Autodesk Fusion 360 part; units mm, degrees
(part 7 of 7)
  line L820 (63.0336, -72.9522) -> (63.1893, -72.6515)
  line L821 (63.1893, -72.6515) -> (63.3708, -72.7431)
  line L822 (63.3708, -72.7431) -> (63.5541, -72.8309)
  line L823 (63.5541, -72.8309) -> (63.7392, -72.9149)
  line L824 (63.7392, -72.9149) -> (63.9261, -72.995)
  line L825 (63.9261, -72.995) -> (63.7958, -73.3076)
  line L826 (63.7958, -73.3076) -> (63.771, -73.385)
  line L827 (63.771, -73.385) -> (63.7515, -73.4645)
  line L828 (63.7515, -73.4645) -> (63.7355, -73.5455)
  line L829 (63.7355, -73.5455) -> (63.7225, -73.6277)
  line L830 (63.7225, -73.6277) -> (63.7121, -73.7109)
  line L831 (63.7121, -73.7109) -> (63.704, -73.795)
  line L832 (63.704, -73.795) -> (63.6981, -73.8799)
  line L833 (63.6981, -73.8799) -> (63.6944, -73.9656)
  line L834 (63.6944, -73.9656) -> (63.6926, -74.0521)
  line L835 (63.6926, -74.0521) -> (63.6927, -74.1391)
  line L836 (63.6927, -74.1391) -> (63.6947, -74.2268)
  line L837 (63.6947, -74.2268) -> (63.6986, -74.3151)
  line L838 (63.6986, -74.3151) -> (63.8305, -74.365)
  line L839 (63.8305, -74.365) -> (63.9631, -74.4133)
  line L840 (63.9631, -74.4133) -> (64.0963, -74.4599)
  line L841 (64.0963, -74.4599) -> (64.156, -74.3947)
  line L842 (64.156, -74.3947) -> (64.2139, -74.3288)
  line L843 (64.2139, -74.3288) -> (64.2699, -74.2622)
  line L844 (64.2699, -74.2622) -> (64.3241, -74.1949)
  line L845 (64.3241, -74.1949) -> (64.3763, -74.1268)
  line L846 (64.3763, -74.1268) -> (64.4264, -74.058)
  line L847 (64.4264, -74.058) -> (64.4743, -73.9883)
  line L848 (64.4743, -73.9883) -> (64.5198, -73.9179)
  line L849 (64.5198, -73.9179) -> (64.5627, -73.8466)
  line L850 (64.5627, -73.8466) -> (64.6025, -73.7743)
  line L851 (64.6025, -73.7743) -> (64.6387, -73.7008)
  line L852 (64.6387, -73.7008) -> (64.6694, -73.6256)
  line L853 (64.6694, -73.6256) -> (64.7705, -73.3024)
  line L854 (64.7705, -73.3024) -> (64.9652, -73.3611)
  line L855 (64.9652, -73.3611) -> (65.161, -73.4157)
  line L856 (65.161, -73.4157) -> (65.3579, -73.4663)
  line L857 (65.3579, -73.4663) -> (65.5558, -73.5128)
  line L858 (65.5558, -73.5128) -> (65.4818, -73.8433)
  line L859 (65.4818, -73.8433) -> (65.4708, -73.9238)
  line L860 (65.4708, -73.9238) -> (65.4654, -74.0055)
  line L861 (65.4654, -74.0055) -> (65.4637, -74.088)
  line L862 (65.4637, -74.088) -> (65.4652, -74.1712)
  line L863 (65.4652, -74.1712) -> (65.4693, -74.255)
  line L864 (65.4693, -74.255) -> (65.476, -74.3392)
  line L865 (65.476, -74.3392) -> (65.485, -74.4238)
  line L866 (65.485, -74.4238) -> (65.4962, -74.5089)
  line L867 (65.4962, -74.5089) -> (65.5094, -74.5943)
  line L868 (65.5094, -74.5943) -> (65.5247, -74.68)
  line L869 (65.5247, -74.68) -> (65.5419, -74.766)
  line L870 (65.5419, -74.766) -> (65.561, -74.8523)
  line L871 (65.561, -74.8523) -> (65.6996, -74.8786)
  line L872 (65.6996, -74.8786) -> (65.8385, -74.9031)
  line L873 (65.8385, -74.9031) -> (65.9778, -74.9258)
  line L874 (65.9778, -74.9258) -> (66.0252, -74.8513)
  line L875 (66.0252, -74.8513) -> (66.0708, -74.7763)
  line L876 (66.0708, -74.7763) -> (66.1145, -74.701)
  line L877 (66.1145, -74.701) -> (66.1562, -74.6253)
  line L878 (66.1562, -74.6253) -> (66.1957, -74.5492)
  line L879 (66.1957, -74.5492) -> (66.2331, -74.4727)
  line L880 (66.2331, -74.4727) -> (66.2682, -74.3958)
  line L881 (66.2682, -74.3958) -> (66.3008, -74.3186)
  line L882 (66.3008, -74.3186) -> (66.3306, -74.2409)
  line L883 (66.3306, -74.2409) -> (66.3573, -74.1628)
  line L884 (66.3573, -74.1628) -> (66.3802, -74.0841)
  line L885 (66.3802, -74.0841) -> (66.3973, -74.0047)
  line L886 (66.3973, -74.0047) -> (66.4408, -73.6689)
  line L887 (66.4408, -73.6689) -> (66.6427, -73.6929)
  line L888 (66.6427, -73.6929) -> (66.845, -73.7127)
  line L889 (66.845, -73.7127) -> (67.0477, -73.7283)
  line L890 (67.0477, -73.7283) -> (67.2507, -73.7397)
  line L891 (67.2507, -73.7397) -> (67.2352, -74.078)
  line L892 (67.2352, -74.078) -> (67.2383, -74.1592)
  line L893 (67.2383, -74.1592) -> (67.2472, -74.2406)
  line L894 (67.2472, -74.2406) -> (67.2599, -74.3222)
  line L895 (67.2599, -74.3222) -> (67.2757, -74.4039)
  line L896 (67.2757, -74.4039) -> (67.2944, -74.4856)
  line L897 (67.2944, -74.4856) -> (67.3156, -74.5674)
  line L898 (67.3156, -74.5674) -> (67.3391, -74.6492)
  line L899 (67.3391, -74.6492) -> (67.3649, -74.731)
  line L900 (67.3649, -74.731) -> (67.3928, -74.8128)
  line L901 (67.3928, -74.8128) -> (67.4227, -74.8946)
  line L902 (67.4227, -74.8946) -> (67.4546, -74.9763)
  line L903 (67.4546, -74.9763) -> (67.4884, -75.058)
  line L904 (67.4884, -75.058) -> (67.6295, -75.0598)
  line L905 (67.6295, -75.0598) -> (67.7705, -75.0598)
  line L906 (67.7705, -75.0598) -> (67.9116, -75.058)
  line L907 (67.9116, -75.058) -> (67.9454, -74.9763)
  line L908 (67.9454, -74.9763) -> (67.9773, -74.8946)
  line L909 (67.9773, -74.8946) -> (68.0072, -74.8128)
  line L910 (68.0072, -74.8128) -> (68.0351, -74.731)
  line L911 (68.0351, -74.731) -> (68.0609, -74.6492)
  line L912 (68.0609, -74.6492) -> (68.0844, -74.5674)
  line L913 (68.0844, -74.5674) -> (68.1056, -74.4856)
  line L914 (68.1056, -74.4856) -> (68.1243, -74.4039)
  line L915 (68.1243, -74.4039) -> (68.1401, -74.3222)
  line L916 (68.1401, -74.3222) -> (68.1528, -74.2406)
  line L917 (68.1528, -74.2406) -> (68.1617, -74.1592)
  line L918 (68.1617, -74.1592) -> (68.1648, -74.078)
  line L919 (68.1648, -74.078) -> (68.1493, -73.7397)
  line L920 (68.1493, -73.7397) -> (68.3523, -73.7283)
  line L921 (68.3523, -73.7283) -> (68.555, -73.7127)
  line L922 (68.555, -73.7127) -> (68.7573, -73.6929)
  line L923 (68.7573, -73.6929) -> (68.9592, -73.6689)
  line L924 (68.9592, -73.6689) -> (69.0027, -74.0047)
  line L925 (69.0027, -74.0047) -> (69.0198, -74.0841)
  line L926 (69.0198, -74.0841) -> (69.0427, -74.1628)
  line L927 (69.0427, -74.1628) -> (69.0694, -74.2409)
  line L928 (69.0694, -74.2409) -> (69.0992, -74.3186)
  line L929 (69.0992, -74.3186) -> (69.1318, -74.3958)
  line L930 (69.1318, -74.3958) -> (69.1669, -74.4727)
  line L931 (69.1669, -74.4727) -> (69.2043, -74.5492)
  line L932 (69.2043, -74.5492) -> (69.2438, -74.6253)
  line L933 (69.2438, -74.6253) -> (69.2855, -74.701)
  line L934 (69.2855, -74.701) -> (69.3292, -74.7763)
  line L935 (69.3292, -74.7763) -> (69.3748, -74.8513)
  line L936 (69.3748, -74.8513) -> (69.4222, -74.9258)
  line L937 (69.4222, -74.9258) -> (69.5615, -74.9031)
  line L938 (69.5615, -74.9031) -> (69.7004, -74.8786)
  line L939 (69.7004, -74.8786) -> (69.839, -74.8523)
  line L940 (69.839, -74.8523) -> (69.8581, -74.766)
  line L941 (69.8581, -74.766) -> (69.8753, -74.68)
  line L942 (69.8753, -74.68) -> (69.8906, -74.5943)
  line L943 (69.8906, -74.5943) -> (69.9038, -74.5089)
  line L944 (69.9038, -74.5089) -> (69.915, -74.4238)
  line L945 (69.915, -74.4238) -> (69.924, -74.3392)
  line L946 (69.924, -74.3392) -> (69.9307, -74.255)
  line L947 (69.9307, -74.255) -> (69.9348, -74.1712)
  line L948 (69.9348, -74.1712) -> (69.9363, -74.088)
  line L949 (69.9363, -74.088) -> (69.9346, -74.0055)
  line L950 (69.9346, -74.0055) -> (69.9292, -73.9238)
  line L951 (69.9292, -73.9238) -> (69.9182, -73.8433)
  line L952 (69.9182, -73.8433) -> (69.8442, -73.5128)
  line L953 (69.8442, -73.5128) -> (70.0421, -73.4663)
  line L954 (70.0421, -73.4663) -> (70.239, -73.4157)
  line L955 (70.239, -73.4157) -> (70.4348, -73.3611)
  line L956 (70.4348, -73.3611) -> (70.6295, -73.3024)
  line L957 (70.6295, -73.3024) -> (70.7306, -73.6256)
  line L958 (70.7306, -73.6256) -> (70.7613, -73.7008)
  line L959 (70.7613, -73.7008) -> (70.7975, -73.7743)
  line L960 (70.7975, -73.7743) -> (70.8373, -73.8466)
  line L961 (70.8373, -73.8466) -> (70.8802, -73.9179)
  line L962 (70.8802, -73.9179) -> (70.9257, -73.9883)
  line L963 (70.9257, -73.9883) -> (70.9736, -74.058)
  line L964 (70.9736, -74.058) -> (71.0237, -74.1268)
  line L965 (71.0237, -74.1268) -> (71.0759, -74.1949)
  line L966 (71.0759, -74.1949) -> (71.1301, -74.2622)
  line L967 (71.1301, -74.2622) -> (71.1861, -74.3288)
  line L968 (71.1861, -74.3288) -> (71.244, -74.3947)
  line L969 (71.244, -74.3947) -> (71.3037, -74.4599)
  line L970 (71.3037, -74.4599) -> (71.4369, -74.4133)
  line L971 (71.4369, -74.4133) -> (71.5695, -74.365)
  line L972 (71.5695, -74.365) -> (71.7014, -74.3151)
  line L973 (71.7014, -74.3151) -> (71.7053, -74.2268)
  line L974 (71.7053, -74.2268) -> (71.7073, -74.1391)
  line L975 (71.7073, -74.1391) -> (71.7074, -74.0521)
  line L976 (71.7074, -74.0521) -> (71.7056, -73.9656)
  line L977 (71.7056, -73.9656) -> (71.7019, -73.8799)
  line L978 (71.7019, -73.8799) -> (71.696, -73.795)
  line L979 (71.696, -73.795) -> (71.6879, -73.7109)
  line L980 (71.6879, -73.7109) -> (71.6775, -73.6277)
  line L981 (71.6775, -73.6277) -> (71.6645, -73.5455)
  line L982 (71.6645, -73.5455) -> (71.6485, -73.4645)
  line L983 (71.6485, -73.4645) -> (71.629, -73.385)
  line L984 (71.629, -73.385) -> (71.6042, -73.3076)
  line L985 (71.6042, -73.3076) -> (71.4739, -72.995)
  line L986 (71.4739, -72.995) -> (71.6608, -72.9149)
  line L987 (71.6608, -72.9149) -> (71.8459, -72.8309)
  line L988 (71.8459, -72.8309) -> (72.0292, -72.7431)
  line L989 (72.0292, -72.7431) -> (72.2107, -72.6515)
  line L990 (72.2107, -72.6515) -> (72.3664, -72.9522)
  line L991 (72.3664, -72.9522) -> (72.4097, -73.0209)
  line L992 (72.4097, -73.0209) -> (72.4581, -73.087)
  line L993 (72.4581, -73.087) -> (72.5099, -73.1513)
  line L994 (72.5099, -73.1513) -> (72.5645, -73.2141)
  line L995 (72.5645, -73.2141) -> (72.6215, -73.2756)
  line L996 (72.6215, -73.2756) -> (72.6808, -73.3358)
  line L997 (72.6808, -73.3358) -> (72.7421, -73.3949)
  line L998 (72.7421, -73.3949) -> (72.8053, -73.4528)
  line L999 (72.8053, -73.4528) -> (72.8704, -73.5097)
  line L1000 (72.8704, -73.5097) -> (72.9372, -73.5656)
  line L1001 (72.9372, -73.5656) -> (73.0056, -73.6204)
  line L1002 (73.0056, -73.6204) -> (73.0757, -73.6743)
  line L1003 (73.0757, -73.6743) -> (73.1988, -73.6053)
  line L1004 (73.1988, -73.6053) -> (73.321, -73.5347)
  line L1005 (73.321, -73.5347) -> (73.4423, -73.4626)
  line L1006 (73.4423, -73.4626) -> (73.4307, -73.375)
  line L1007 (73.4307, -73.375) -> (73.4174, -73.2883)
  line L1008 (73.4174, -73.2883) -> (73.4025, -73.2025)
  line L1009 (73.4025, -73.2025) -> (73.3857, -73.1178)
  line L1010 (73.3857, -73.1178) -> (73.3671, -73.034)
  line L1011 (73.3671, -73.034) -> (73.3466, -72.9514)
  line L1012 (73.3466, -72.9514) -> (73.3241, -72.87)
  line L1013 (73.3241, -72.87) -> (73.2993, -72.7898)
  line L1014 (73.2993, -72.7898) -> (73.2723, -72.7112)
  line L1015 (73.2723, -72.7112) -> (73.2425, -72.6342)
  line L1016 (73.2425, -72.6342) -> (73.2095, -72.5592)
  line L1017 (73.2095, -72.5592) -> (73.1716, -72.4874)
  line L1018 (73.1716, -72.4874) -> (72.989, -72.2021)
  line L1019 (72.989, -72.2021) -> (73.1591, -72.0908)
  line L1020 (73.1591, -72.0908) -> (73.3268, -71.9759)
  line L1021 (73.3268, -71.9759) -> (73.4921, -71.8576)
  line L1022 (73.4921, -71.8576) -> (73.6549, -71.7358)
  line L1023 (73.6549, -71.7358) -> (73.8605, -72.005)
  line L1024 (73.8605, -72.005) -> (73.9151, -72.0651)
  line L1025 (73.9151, -72.0651) -> (73.9742, -72.1218)
  line L1026 (73.9742, -72.1218) -> (74.0364, -72.1761)
  line L1027 (74.0364, -72.1761) -> (74.101, -72.2285)
  line L1028 (74.101, -72.2285) -> (74.1679, -72.2791)
  line L1029 (74.1679, -72.2791) -> (74.2367, -72.3281)
  line L1030 (74.2367, -72.3281) -> (74.3073, -72.3757)
  line L1031 (74.3073, -72.3757) -> (74.3796, -72.4218)
  line L1032 (74.3796, -72.4218) -> (74.4536, -72.4665)
  line L1033 (74.4536, -72.4665) -> (74.5291, -72.5099)
  line L1034 (74.5291, -72.5099) -> (74.606, -72.5521)
  line L1035 (74.606, -72.5521) -> (74.6844, -72.5929)
  line L1036 (74.6844, -72.5929) -> (74.7936, -72.5036)
  line L1037 (74.7936, -72.5036) -> (74.9017, -72.4129)
  line L1038 (74.9017, -72.4129) -> (75.0086, -72.3208)
  line L1039 (75.0086, -72.3208) -> (74.982, -72.2366)
  line L1040 (74.982, -72.2366) -> (74.9539, -72.1535)
  line L1041 (74.9539, -72.1535) -> (74.9242, -72.0716)
  line L1042 (74.9242, -72.0716) -> (74.893, -71.991)
  line L1043 (74.893, -71.991) -> (74.8602, -71.9118)
  line L1044 (74.8602, -71.9118) -> (74.8256, -71.834)
  line L1045 (74.8256, -71.834) -> (74.7893, -71.7577)
  line L1046 (74.7893, -71.7577) -> (74.751, -71.6831)
  line L1047 (74.751, -71.6831) -> (74.7107, -71.6103)
  line L1048 (74.7107, -71.6103) -> (74.668, -71.5397)
  line L1049 (74.668, -71.5397) -> (74.6225, -71.4716)
  line L1050 (74.6225, -71.4716) -> (74.5727, -71.4074)
  line L1051 (74.5727, -71.4074) -> (74.3433, -71.1582)
  line L1052 (74.3433, -71.1582) -> (74.4915, -71.019)
  line L1053 (74.4915, -71.019) -> (74.6367, -70.8767)
  line L1054 (74.6367, -70.8767) -> (74.779, -70.7315)
  line L1055 (74.779, -70.7315) -> (74.9182, -70.5833)
  line L1056 (74.9182, -70.5833) -> (75.1674, -70.8127)
  line L1057 (75.1674, -70.8127) -> (75.2316, -70.8625)
  line L1058 (75.2316, -70.8625) -> (75.2997, -70.908)
  line L1059 (75.2997, -70.908) -> (75.3703, -70.9507)
  line L1060 (75.3703, -70.9507) -> (75.4431, -70.991)
  line L1061 (75.4431, -70.991) -> (75.5177, -71.0293)
  line L1062 (75.5177, -71.0293) -> (75.594, -71.0656)
  line L1063 (75.594, -71.0656) -> (75.6718, -71.1002)
  line L1064 (75.6718, -71.1002) -> (75.751, -71.133)
  line L1065 (75.751, -71.133) -> (75.8316, -71.1642)
  line L1066 (75.8316, -71.1642) -> (75.9135, -71.1939)
  line L1067 (75.9135, -71.1939) -> (75.9966, -71.222)
  line L1068 (75.9966, -71.222) -> (76.0808, -71.2486)
  line L1069 (76.0808, -71.2486) -> (76.1729, -71.1417)
  line L1070 (76.1729, -71.1417) -> (76.2636, -71.0336)
  line L1071 (76.2636, -71.0336) -> (76.3529, -70.9244)
  line L1072 (76.3529, -70.9244) -> (76.3121, -70.846)
  line L1073 (76.3121, -70.846) -> (76.2699, -70.7691)
  line L1074 (76.2699, -70.7691) -> (76.2265, -70.6936)
  line L1075 (76.2265, -70.6936) -> (76.1818, -70.6196)
  line L1076 (76.1818, -70.6196) -> (76.1357, -70.5473)
  line L1077 (76.1357, -70.5473) -> (76.0881, -70.4767)
  line L1078 (76.0881, -70.4767) -> (76.0391, -70.4079)
  line L1079 (76.0391, -70.4079) -> (75.9885, -70.341)
  line L1080 (75.9885, -70.341) -> (75.9361, -70.2764)
  line L1081 (75.9361, -70.2764) -> (75.8818, -70.2142)
  line L1082 (75.8818, -70.2142) -> (75.8251, -70.1551)
  line L1083 (75.8251, -70.1551) -> (75.765, -70.1005)
  line L1084 (75.765, -70.1005) -> (75.4958, -69.8949)
  line L1085 (75.4958, -69.8949) -> (75.6176, -69.7321)
  line L1086 (75.6176, -69.7321) -> (75.7359, -69.5668)
  line L1087 (75.7359, -69.5668) -> (75.8508, -69.3991)
  line L1088 (75.8508, -69.3991) -> (75.9621, -69.229)
  line L1089 (75.9621, -69.229) -> (76.2474, -69.4116)
  line L1090 (76.2474, -69.4116) -> (76.3192, -69.4495)
  line L1091 (76.3192, -69.4495) -> (76.3942, -69.4825)
  line L1092 (76.3942, -69.4825) -> (76.4712, -69.5123)
  line L1093 (76.4712, -69.5123) -> (76.5498, -69.5393)
  line L1094 (76.5498, -69.5393) -> (76.63, -69.5641)
  line L1095 (76.63, -69.5641) -> (76.7114, -69.5866)
  line L1096 (76.7114, -69.5866) -> (76.794, -69.6071)
  line L1097 (76.794, -69.6071) -> (76.8778, -69.6257)
  line L1098 (76.8778, -69.6257) -> (76.9625, -69.6425)
  line L1099 (76.9625, -69.6425) -> (77.0483, -69.6574)
  line L1100 (77.0483, -69.6574) -> (77.135, -69.6707)
  line L1101 (77.135, -69.6707) -> (77.2226, -69.6823)
  line L1102 (77.2226, -69.6823) -> (77.2947, -69.561)
  line L1103 (77.2947, -69.561) -> (77.3653, -69.4388)
  line L1104 (77.3653, -69.4388) -> (77.4343, -69.3157)
  line L1105 (77.4343, -69.3157) -> (77.3804, -69.2456)
  line L1106 (77.3804, -69.2456) -> (77.3256, -69.1772)
  line L1107 (77.3256, -69.1772) -> (77.2697, -69.1104)
  line L1108 (77.2697, -69.1104) -> (77.2128, -69.0453)
  line L1109 (77.2128, -69.0453) -> (77.1549, -68.9821)
  line L1110 (77.1549, -68.9821) -> (77.0958, -68.9208)
  line L1111 (77.0958, -68.9208) -> (77.0356, -68.8615)
  line L1112 (77.0356, -68.8615) -> (76.9741, -68.8045)
  line L1113 (76.9741, -68.8045) -> (76.9113, -68.7499)
  line L1114 (76.9113, -68.7499) -> (76.847, -68.6981)
  line L1115 (76.847, -68.6981) -> (76.7809, -68.6497)
  line L1116 (76.7809, -68.6497) -> (76.7122, -68.6064)
  line L1117 (76.7122, -68.6064) -> (76.4115, -68.4507)
  line L1118 (76.4115, -68.4507) -> (76.5031, -68.2692)
  line L1119 (76.5031, -68.2692) -> (76.5909, -68.0859)
  line L1120 (76.5909, -68.0859) -> (76.6749, -67.9008)
  line L1121 (76.6749, -67.9008) -> (76.755, -67.7139)
  line L1122 (76.755, -67.7139) -> (77.0676, -67.8442)
  line L1123 (77.0676, -67.8442) -> (77.145, -67.869)
  line L1124 (77.145, -67.869) -> (77.2245, -67.8885)
  line L1125 (77.2245, -67.8885) -> (77.3055, -67.9045)
  line L1126 (77.3055, -67.9045) -> (77.3877, -67.9175)
  line L1127 (77.3877, -67.9175) -> (77.4709, -67.9279)
  line L1128 (77.4709, -67.9279) -> (77.555, -67.936)
  line L1129 (77.555, -67.936) -> (77.6399, -67.9419)
  line L1130 (77.6399, -67.9419) -> (77.7256, -67.9456)
  line L1131 (77.7256, -67.9456) -> (77.8121, -67.9474)
  line L1132 (77.8121, -67.9474) -> (77.8991, -67.9473)
  line L1133 (77.8991, -67.9473) -> (77.9868, -67.9453)
  line L1134 (77.9868, -67.9453) -> (78.0751, -67.9414)
  line L1135 (78.0751, -67.9414) -> (78.125, -67.8095)
  line L1136 (78.125, -67.8095) -> (78.1733, -67.6769)
  line L1137 (78.1733, -67.6769) -> (78.2199, -67.5437)
  line L1138 (78.2199, -67.5437) -> (78.1547, -67.484)
  line L1139 (78.1547, -67.484) -> (78.0888, -67.4261)
  line L1140 (78.0888, -67.4261) -> (78.0222, -67.3701)
  line L1141 (78.0222, -67.3701) -> (77.9549, -67.3159)
  line L1142 (77.9549, -67.3159) -> (77.8868, -67.2637)
  line L1143 (77.8868, -67.2637) -> (77.818, -67.2136)
  line L1144 (77.818, -67.2136) -> (77.7483, -67.1657)
  line L1145 (77.7483, -67.1657) -> (77.6779, -67.1202)
  line L1146 (77.6779, -67.1202) -> (77.6066, -67.0773)
  line L1147 (77.6066, -67.0773) -> (77.5343, -67.0375)
  line L1148 (77.5343, -67.0375) -> (77.4608, -67.0013)
  line L1149 (77.4608, -67.0013) -> (77.3856, -66.9706)
  line L1150 (77.3856, -66.9706) -> (77.0624, -66.8695)
  line L1151 (77.0624, -66.8695) -> (77.1211, -66.6748)
  line L1152 (77.1211, -66.6748) -> (77.1757, -66.479)
  line L1153 (77.1757, -66.479) -> (77.2263, -66.2821)
  line L1154 (77.2263, -66.2821) -> (77.2728, -66.0842)
  line L1155 (77.2728, -66.0842) -> (77.6033, -66.1582)
  line L1156 (77.6033, -66.1582) -> (77.6838, -66.1692)
  line L1157 (77.6838, -66.1692) -> (77.7655, -66.1746)
  line L1158 (77.7655, -66.1746) -> (77.848, -66.1763)
  line L1159 (77.848, -66.1763) -> (77.9312, -66.1748)
  line L1160 (77.9312, -66.1748) -> (78.015, -66.1707)
  line L1161 (78.015, -66.1707) -> (78.0992, -66.164)
  line L1162 (78.0992, -66.164) -> (78.1838, -66.155)
  line L1163 (78.1838, -66.155) -> (78.2689, -66.1438)
  line L1164 (78.2689, -66.1438) -> (78.3543, -66.1306)
  line L1165 (78.3543, -66.1306) -> (78.44, -66.1153)
  line L1166 (78.44, -66.1153) -> (78.526, -66.0981)
  line L1167 (78.526, -66.0981) -> (78.6123, -66.079)
  line L1168 (78.6123, -66.079) -> (78.6386, -65.9404)
  line L1169 (78.6386, -65.9404) -> (78.6631, -65.8015)
  line L1170 (78.6631, -65.8015) -> (78.6858, -65.6622)
  line L1171 (78.6858, -65.6622) -> (78.6113, -65.6148)
  line L1172 (78.6113, -65.6148) -> (78.5363, -65.5692)
  line L1173 (78.5363, -65.5692) -> (78.461, -65.5255)
  line L1174 (78.461, -65.5255) -> (78.3853, -65.4838)
  line L1175 (78.3853, -65.4838) -> (78.3092, -65.4443)
  line L1176 (78.3092, -65.4443) -> (78.2327, -65.4069)
  line L1177 (78.2327, -65.4069) -> (78.1558, -65.3718)
  line L1178 (78.1558, -65.3718) -> (78.0786, -65.3392)
  line L1179 (78.0786, -65.3392) -> (78.0009, -65.3094)
  line L1180 (78.0009, -65.3094) -> (77.9228, -65.2827)
  line L1181 (77.9228, -65.2827) -> (77.8441, -65.2598)
  line L1182 (77.8441, -65.2598) -> (77.7647, -65.2427)
  line L1183 (77.7647, -65.2427) -> (77.4289, -65.1992)
  line L1184 (77.4289, -65.1992) -> (77.4529, -64.9973)
  line L1185 (77.4529, -64.9973) -> (77.4727, -64.795)
  line L1186 (77.4727, -64.795) -> (77.4883, -64.5923)
  line L1187 (77.4883, -64.5923) -> (77.4997, -64.3893)
  circle A0 centre (67.7, -63.94) radius 1.6
extrude "Extrude1''''" add sketch "Sketch1 (5)" along normal blind 2 separate body makes body 11 in component "CT dial wheel (tool body)"
component "CT sprocket pinion (tool body)" placed x (1, 0, 0) y (0, 1, 0) z (0, 0, 1) at (0, 0, 0)
component "CT idler 1" placed x (1, 0, 0) y (0, 1, 0) z (0, 0, 1) at (0, 0, 0)
component "CT idler 2" placed x (1, 0, 0) y (0, 1, 0) z (0, 0, 1) at (0, 0, 0)
component "CT idler 3" placed x (1, 0, 0) y (0, 1, 0) z (0, 0, 1) at (0, 0, 0)
component "CT dial wheel (tool body)" placed x (1, 0, 0) y (0, 1, 0) z (0, 0, 1) at (0, 0, 0)
equation "ct_module = 0.6 mm" comment "Counter train: gear module"
equation "ct_pressure_angle = 20.0 deg" comment "Counter train: pressure angle"
equation "ct_pinion_teeth = 12" comment "Counter train: teeth on every pinion"
equation "ct_wheel1_teeth = 32" comment "Counter train: idler 1 wheel (meshes sprocket pinion)"
equation "ct_wheel2_teeth = 30" comment "Counter train: idler 2 wheel"
equation "ct_wheel3_teeth = 30" comment "Counter train: idler 3 wheel"
equation "ct_wheel4_teeth = 36" comment "Counter train: dial wheel"
equation "ct_thinning = 0.1 mm" comment "Counter train: tooth thinning per gear (backlash share)"
equation "ct_pinion_shift = 0.4" comment "Counter train: pinion profile shift x (wheels get -x)"
equation "ct_pinion_tip_reduction = 0.1 mm" comment "Counter train: pinion tip shave (radial)"
equation "ct_wheel_tip_reduction = 0.04 mm" comment "Counter train: wheel tip shave (radial)"
equation "ct_sprocket_x = 73.2 mm" comment "Counter train: sprocket axis X (fixed)"
equation "ct_sprocket_y = -45.21 mm" comment "Counter train: sprocket axis Y (fixed)"
equation "ct_dial_x = 67.7 mm" comment "Counter train: dial axis X (fixed)"
equation "ct_dial_y = -63.94 mm" comment "Counter train: dial axis Y (fixed)"
equation "ct_idler1_angle = -90.74 deg" comment "Counter train: direction sprocket -> idler 1"
equation "ct_idler2_angle = -164.0 deg" comment "Counter train: direction idler 1 -> idler 2"
equation "ct_idler3_elbow = 1" comment "Counter train: idler 3 solution, 1 or -1"
equation "ct_face_width = 2.0 mm" comment "Counter train: gear face width"
equation "ct_layer_gap = 0.2 mm" comment "Counter train: axial gap between gear layers"
equation "ct_base_z = 36.8 mm" comment "Counter train: underside of idler 1 wheel"
equation "ct_clearance = 0.3 mm" comment "Counter train: minimum gap to non-meshing parts"
equation "ct_bore1 = 4.4 mm" comment "Counter train: idler 1 bore"
equation "ct_bore2 = 4.0 mm" comment "Counter train: idler 2 bore"
equation "ct_bore3 = 3.0 mm" comment "Counter train: idler 3 bore"
equation "ct_bore4 = 3.2 mm" comment "Counter train: dial wheel bore"
named bodies: "CT sprocket pinion (tool body)", "CT idler 1", "CT idler 1 pinion", "CT idler 1 wheel (1)", "CT idler 2", "CT idler 2 pinion", "CT idler 2 wheel (1)", "CT idler 3", "CT idler 3 pinion", "CT idler 3 wheel (1)", "CT dial wheel (tool body)"
